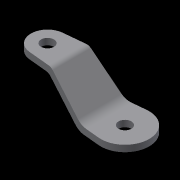
# Autodesk Inventor part: BackConnector
Saved by Autodesk Inventor 2015 (Build 190159000, 159)
## iProperties
Created: 2014-09-27
Part Number: BackConnector
Material: Generic
Document SubType Name: Modeling
Designer: Inventor
Density: 1 g/cm^3
Appearance: Default
Mass: 3.11786 g
Surface Area: 26.1019 cm^2
Volume: 3.11786 cm^3
Author: Inventor
Autodesk Inventor part; units mm, degrees
ref_plane "YZ Plane" through (0, 0, 0) normal (1, 0, 0) x (0, 1, 0)
ref_plane "XY Plane" through (0, 0, 0) normal (0, 0, 1) x (1, 0, 0)
sketch "Body" plane through (0, 0, 0) normal (0, 0, 1) x (1, 0, 0)
  circle A0 centre (0, 0) radius 7.75
  line L0 (0, 0) -> (36, 0) construction
  circle A1 centre (36, 0) radius 11.25
  line L1 (-0.7535, 7.7133) -> (34.9062, 11.1967)
  line L2 (-0.7535, -7.7133) -> (34.9062, -11.1967)
  dimension "SmallDiameter" = 15.5
  dimension "d1" = 36
  dimension "LargeDiameter" = 22.5
  constraints: 6 end point, 4 point on circle, 4 tangent, 2 centre point, 2 coincident, 1 horizontal
  measures "SmallDiameter" diameter of A0
  measures "d1" distance of L0.start L0.end
  measures "LargeDiameter" diameter of A1
extrude "BodyFeature" add sketch "Body" along normal blind 18
sketch "Sketch2" plane through (0, 0, 18) normal (0, 0, 1) x (1, 0, 0)
  arc A0 (-0.7535, 7.7133) -> (-0.7535, -7.7133) centre (0, 0) ccw construction
  line L0 (-0.7535, -7.7133) -> (34.9062, -11.1967) construction
  arc A1 (34.9062, -11.1967) -> (34.9062, 11.1967) centre (36, 0) ccw construction
  line L1 (34.9062, 11.1967) -> (-0.7535, 7.7133) construction
hole "BodyHolesFeature" at (0, 0, 18) at (36, 0, 18) direction (0, 0, -1) diameter 6 end through all
ref_plane "SideProfilePlane" through (0, 12, 0) normal (0, 1, 0) x (-1, 0, 0)
sketch "SideProfile" plane through (0, 12, 0) normal (0, 1, 0) x (-1, 0, 0)
  line L0 (7.75, 18) -> (0.7535, 18) construction
  line L1 (7.75, 18) -> (7.75, 15)
  line L2 (7.75, 15) -> (-9.25, 15)
  line L3 (-9.25, 15) -> (-24.75, 0)
  line L4 (-24.75, 0) -> (-47.25, 0)
  line L5 (-34.9062, 0) -> (0.7535, 0) construction
  line L6 (-47.25, 0) -> (-47.25, 18) construction
  line L7 (-34.9062, 18) -> (-47.25, 18) construction
  line L8 (-34.9062, 18) -> (0.7535, 18) construction
  line L9 (-25.9639, 3) -> (-10.4639, 18)
  line L10 (-47.25, 3) -> (-25.9639, 3)
  line L11 (-47.25, 0) -> (-47.25, 3)
  line L12 (7.75, 18) -> (-10.4639, 18)
  dimension "Thickness" = 3
  dimension "d15" = 3
  dimension "d16" = 3
  dimension "d17" = 17
  dimension "d18" = 22.5
  constraints: 16 end point, 4 collinear, 1 horizontal, 1 parallel, 1 vertical
  measures "Thickness" distance of L0.start L1.end
  measures "d15" distance between parallel lines of L3 L9
  measures "d16" distance of L10.start L4.end
  measures "d17" distance of L1.end L2.end
  measures "d18" distance of L3.end L4.end
extrude "SideProfileFeature" cut sketch "SideProfile" against normal through all keep common part
fillet "SmallFilletFeature" radius 3 2 edges at (9.25, 0, 15) (10.4639, 0, 18)
fillet "LargeFilletFeature" radius 6 2 edges at (24.75, 0, 0) (25.9639, 0, 3)
equation "\"d15\" = Thickness"
equation "\"d16\" = Thickness"
equation "\"d18\" = LargeDiameter"
